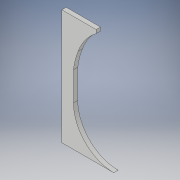
# Autodesk Inventor part: Part3
Saved by Autodesk Inventor 2018 (Build 220112000, 112)
## iProperties
Created: 2020-02-01
Part Number: Part3
Material: Generic
Document SubType Name: Modeling
Designer: Weeb No1
Density: 1 g/cm^3
Appearance: Default
Author: Weeb No1
Autodesk Inventor part; units mm, degrees
ref_plane "YZ Plane" through (0, 0, 0) normal (1, 0, 0) x (0, 1, 0)
ref_plane "XZ Plane" through (0, 0, 0) normal (0, 1, 0) x (-1, 0, 0)
ref_plane "XY Plane" through (0, 0, 0) normal (0, 0, 1) x (1, 0, 0)
sketch "Sketch1" plane through (0, 0, 0) normal (0, 0, 1) x (1, 0, 0)
  line L0 (0, 0) -> (609.6, 0) construction
  line L1 (609.6, 0) -> (609.6, 209.55)
  line L2 (609.6, 209.55) -> (0, 209.55) construction
  line L3 (0, 209.55) -> (0, 0) construction
  line L4 (0, 0) -> (304.8, 0) construction
  line L5 (304.8, 0) -> (304.8, 165.1) construction
  line L6 (304.8, 165.1) -> (0, 165.1) construction
  line L7 (0, 165.1) -> (0, 0) construction
  line L8 (0, 0) -> (165.1, 0) construction
  line L9 (165.1, 0) -> (165.1, 304.8) construction
  line L10 (165.1, 304.8) -> (0, 304.8) construction
  line L11 (0, 304.8) -> (0, 0) construction
  line L12 (0, 0) -> (177.8, 0) construction
  line L13 (177.8, 0) -> (177.8, 177.8) construction
  line L14 (177.8, 177.8) -> (0, 177.8) construction
  line L15 (0, 177.8) -> (0, 0) construction
  circle A0 centre (177.8, 177.8) radius 12.7
  line L16 (177.8, 177.8) -> (165.1, 177.8)
  line L17 (177.8, 177.8) -> (177.8, 165.1)
  line L18 (177.8, 177.8) -> (168.8197, 168.8197)
  line L19 (177.8, 177.8) -> (190.5, 177.8) construction
  line L20 (168.8197, 168.8197) -> (52.0764, 52.0764) construction
  line L21 (168.8197, 168.8197) -> (333.9197, 168.8197) construction
  line L22 (177.8, 165.1) -> (177.8, 0) construction
  line L23 (165.1, 177.8) -> (0, 177.8) construction
  arc A1 (0, 177.8) -> (177.8, 0) centre (177.8, 177.8) ccw
  line L24 (177.8, 177.8) -> (355.6, 177.8) construction
  line L25 (355.6, 177.8) -> (355.6, 193.675)
  line L26 (355.6, 193.675) -> (177.8, 193.675) construction
  line L27 (177.8, 193.675) -> (177.8, 177.8) construction
  circle A2 centre (355.6, 193.675) radius 12.7
  line L28 (355.6, 193.675) -> (482.6, 193.675) construction
  line L29 (482.6, 209.55) -> (355.6, 209.55) construction
  line L30 (355.6, 209.55) -> (355.6, 193.675) construction
  line L31 (177.8, 0) -> (609.6, 0)
  line L32 (177.8, 165.1) -> (355.6, 180.975)
  line L33 (165.1, 177.8) -> (165.1, 304.8) construction
  line L34 (165.1, 304.8) -> (241.3, 304.8) construction
  circle A3 centre (241.3, 304.8) radius 76.2
  circle A4 centre (177.8, 228.6) radius 12.7
  line L35 (177.8, 177.8) -> (177.8, 228.6)
  line L36 (0, 177.8) -> (0, 304.8)
  line L37 (241.3, 304.8) -> (195.4417, 365.656) construction
  line L38 (241.3, 304.8) -> (317.5, 304.8) construction
  line L39 (195.4417, 365.656) -> (354.1917, 365.656) construction
  line L40 (195.4417, 365.656) -> (99.9036, 492.4394) construction
  line L41 (195.4417, 365.656) -> (354.1917, 365.656) construction
  line L42 (165.1, 304.8) -> (0, 304.8) construction
  line L43 (241.3, 304.8) -> (169.6954, 330.8619) construction
  line L44 (241.3, 304.8) -> (317.5, 304.8) construction
  line L45 (169.6954, 330.8619) -> (20.5192, 385.1576) construction
  line L46 (177.8, 0) -> (408.0964, 0) construction
  line L47 (241.3, 304.8) -> (317.5, 304.8) construction
  line L48 (241.3, 304.8) -> (175.3089, 342.9) construction
  line L49 (241.3, 304.8) -> (317.5, 304.8) construction
  line L50 (175.3089, 342.9) -> (37.8273, 422.275) construction
  arc A5 (99.9036, 492.4394) -> (20.5192, 385.1576) centre (241.3, 304.8) ccw
  arc A6 (37.8273, 422.275) -> (0, 304.8) centre (330.4977, 263.2064) ccw
  line L51 (0, 177.8) -> (0, 304.8)
  line L52 (190.5, 177.8) -> (393.7, 177.8) construction
  line L53 (609.6, 0) -> (-50.8, 0)
  line L54 (-50.8, 0) -> (-50.8, 508)
  line L55 (177.8, 0) -> (-50.8, 0)
  line L56 (-50.8, 492.4394) -> (-50.8, 508)
  line L57 (-50.8, 508) -> (99.9036, 508)
  line L58 (99.9036, 508) -> (99.9036, 492.4394)
  line L59 (355.6, 180.975) -> (609.6, 209.55)
  point P0 (165.2751, 230.7014)
  point P1 (172.7151, 216.9624)
  dimension "d16" = 25.4
  dimension "d0" = 609.6
  dimension "d1" = 209.55
  dimension "d2" = 304.8
  dimension "d3" = 165.1
  dimension "d4" = 165.1
  dimension "d5" = 304.8
  dimension "d6" = 177.8
  dimension "d7" = 177.8
  dimension "d8" = 25.4
  dimension "d9" = 12.7
  dimension "d10" = 135
  dimension "d11" = 165.1
  dimension "d12" = 135
  dimension "d13" = 165.1
  dimension "d14" = 177.8
  dimension "d15" = 15.875
  dimension "d17" = 127
  dimension "d20" = 127
  dimension "d21" = 76.2
  dimension "d22" = 152.4
  dimension "d23" = 25.4
  dimension "d24" = 50.8
  dimension "d25" = 127
  dimension "d26" = 127
  dimension "d33" = 158.75
  dimension "d34" = 127
  dimension "d35" = 160
  dimension "d36" = 158.75
  dimension "d37" = 180
  dimension "d45" = 150
  dimension "d46" = 158.75
  dimension "d47" = 180
  dimension "d72" = 660.4
  dimension "d73" = 508
  dimension "d74" = 90
  dimension "d77" = 150.7036
  dimension "d78" = 15.5606
  constraints: 120 end point, 19 horizontal, 16 point on circle, 12 parallel, 7 collinear, 6 centre point, 6 equal length, 6 perpendicular, 5 coincident, 5 point on line, 1 vertical, 1 vertical alignment, 2 other
  measures "d0" distance of L2.end L1.end
  measures "d1" distance of L1.end L0.end
  measures "d2" distance of L6.end L5.end
  measures "d3" distance of L5.end L4.end
  measures "d4" distance of L10.end L9.end
  measures "d5" distance of L9.end L8.end
  measures "d6" distance of L14.end L13.end
  measures "d7" distance of L13.end L12.end
  measures "d8" diameter of A0
  measures "d9" distance of L16.start L18.end
  measures "d10" angle of L18 L19
  measures "d11" distance of L18.end L20.end
  measures "d12" angle of L20 L21
  measures "d13" distance of L17.end L12.end
  measures "d14" distance of L26.end L25.end
  measures "d15" distance of L25.end L24.end
  measures "d17" distance of L29.end L29.start
  measures "d20" distance of L16.end L33.end
  measures "d21" distance of L33.end L34.end
  measures "d22" diameter of A3
  measures "d23" diameter of A4
  measures "d24" distance of L16.start L35.end
  measures "d25" distance of L14.end L36.end
  measures "d26" angle of L38 L37
  measures "d33" distance of L37.end L40.end
  measures "d34" angle of L41 L40
  measures "d35" angle of L44 L43
  measures "d36" distance of L43.end L45.end
  measures "d37" angle of L45 L43
  measures "d45" angle of L49 L48
  measures "d46" distance of L48.end L50.end
  measures "d47" angle of L48 L50
  measures "d72" distance of L0.end L53.end
  measures "d73" distance of L53.end L54.end
  measures "d74" angle of L53 L54
  measures "d77" distance of L54.end L57.end
  measures "d78" distance of L57.end L40.end
extrude "Extrusion2" add sketch "Sketch1" along normal blind 19.05 contours A1 L53 L54 L57 L58 A5 A6 L36
body "Solid2"
